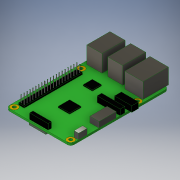
# Autodesk Inventor part: PiB+
Saved by Autodesk Inventor 2016 (Build 200138000, 138)
## iProperties
Created: 2016-08-11
Part Number: PiB+
Material: Generic
Document SubType Name: Modeling
Designer: jfixelle
Density: 1 g/cm^3
Appearance: Smooth - Dark Forest Green
Author: jfixelle
Autodesk Inventor part; units mm, degrees
ref_plane "YZ Plane" through (0, 0, 0) normal (1, 0, 0) x (0, 1, 0)
ref_plane "XZ Plane" through (0, 0, 0) normal (0, 1, 0) x (-1, 0, 0)
ref_plane "XY Plane" through (0, 0, 0) normal (0, 0, 1) x (1, 0, 0)
sketch "Sketch1" plane through (0, 0, 0) normal (0, 1, 0) x (-1, 0, 0)
  line L0 (25, 42.5) -> (-25, 42.5)
  line L1 (-28, 39.5) -> (-28, -39.5)
  line L2 (-25, -42.5) -> (25, -42.5)
  line L3 (28, -39.5) -> (28, 39.5)
  arc A0 (28, 39.5) -> (25, 42.5) centre (25, 39.5) ccw
  arc A1 (25, -42.5) -> (28, -39.5) centre (25, -39.5) ccw
  arc A2 (-28, -39.5) -> (-25, -42.5) centre (-25, -39.5) ccw
  arc A3 (-25, 42.5) -> (-28, 39.5) centre (-25, 39.5) ccw
  line L4 (37.5987, 39) -> (-36.2375, 39) construction
  line L5 (38.7615, -19) -> (-37.8654, -19) construction
  line L6 (-24.5, 52.5969) -> (-24.5, -66.7037) construction
  line L7 (24.5, 56.8992) -> (24.5, -62.5177) construction
  circle A4 centre (24.5, 39) radius 1.4
  circle A5 centre (24.5, -19) radius 1.4
  circle A6 centre (-24.5, -19) radius 1.4
  circle A7 centre (-24.5, 39) radius 1.4
  point P0 (0, 0)
  point P1 (28, 42.5)
  point P2 (-28, -42.5)
  point P3 (28, -42.5)
  dimension "d0" = 85
  dimension "d1" = 56
  dimension "d2" = 42.5
  dimension "d3" = 28
  dimension "d4" = 3
  dimension "d5" = 49
  dimension "d6" = 24.5
  dimension "d7" = 58
  dimension "d8" = 3.5
  dimension "d9" = 2.8
  dimension "d10" = 2.8
  dimension "d11" = 2.8
  dimension "d12" = 2.8
  constraints: 16 end point, 14 point on line, 8 centre point, 8 point on circle, 8 tangent, 3 equal radius, 3 horizontal, 2 parallel, 2 vertical, 1 perpendicular
  measures "d0" distance of point (28, -42.5) point (28, 42.5)
  measures "d1" distance of point (-28, -42.5) point (28, -42.5)
  measures "d2" distance from line of point (0, 0) L2
  measures "d3" distance from line of point (0, 0) L3
  measures "d4" radius of A0
  measures "d5" distance between parallel lines of L6 L7
  measures "d6" distance from line of point (0, 0) L7
  measures "d7" distance between parallel lines of L5 L4
  measures "d8" distance between parallel lines of L0 L4
  measures "d9" diameter of A4
  measures "d10" diameter of A7
  measures "d11" diameter of A6
  measures "d12" diameter of A5
extrude "Extrusion1" add sketch "Sketch1" along normal mid plane 1.65
sketch "Sketch2" plane through (0, 0.825, 0) normal (0, 1, 0) x (1, 0, 0)
  circle A0 centre (-24.5, -39) radius 3.1
  circle A1 centre (-24.5, -39) radius 1.4 projected
  circle A2 centre (-24.5, 19) radius 3.1
  circle A3 centre (24.5, 19) radius 3.1
  circle A4 centre (24.5, -39) radius 3.1
  circle A5 centre (24.5, -39) radius 1.4 projected
  circle A6 centre (24.5, 19) radius 1.4 projected
  circle A7 centre (-24.5, 19) radius 1.4 projected
  point P0 (0, 0)
  dimension "d15" = 6.2
  dimension "d16" = 6.2
  dimension "d17" = 6.2
  dimension "d18" = 6.2
  constraints: 4 centre point, 4 concentric
  measures "d15" diameter of A0
  measures "d16" diameter of A2
  measures "d17" diameter of A3
  measures "d18" diameter of A4
extrude "Extrusion2" add sketch "Sketch2" along normal blind 0.1
mirror "Mirror1" about plane through (0, 0, 0) normal (0, 1, 0) of "Extrusion2"
sketch "Sketch3" plane through (0, 0.825, 0) normal (0, 1, 0) x (1, 0, 0)
  line L0 (-24.5, -35.5) -> (-19.42, -35.5)
  line L1 (-19.42, -35.5) -> (-19.42, 15.3)
  line L2 (-19.42, 15.3) -> (-24.5, 15.3)
  line L3 (-24.5, 15.3) -> (-24.5, -35.5)
  line L4 (-25, -42.5) -> (25, -42.5) projected
  circle A0 centre (-24.5, -39) radius 1.7759
  circle A1 centre (-24.5, -39) radius 1.4 projected
  point P0 (0, 0)
  dimension "d21" = 5.08
  dimension "d22" = 50.8
  dimension "d23" = 7
  dimension "d24" = 0
  constraints: 8 end point, 2 parallel, 1 centre point, 1 concentric, 1 horizontal, 1 perpendicular
  measures "d21" distance of L0.start L0.end
  measures "d22" distance of L0.end L1.end
  measures "d23" distance between parallel lines of L4 L0
  measures "d24" distance from line of A0.centre L3
extrude "Extrusion3" add sketch "Sketch3" along normal blind 1.5 contours L3 L2 L1 L0
sketch "Sketch5" plane through (0, 2.325, 0) normal (0, 1, 0) x (1, 0, 0)
  circle A0 centre (-23.23, -34.23) radius 0.32
  line L0 (-24.5, 15.3) -> (-24.5, -35.5) projected
  line L1 (-24.5, -35.5) -> (-19.42, -35.5) projected
  point P0 (0, 0)
  dimension "d27" = 1.27
  dimension "d28" = 1.27
  dimension "d29" = 0.64
  constraints: 1 centre point
  measures "d27" distance from line of L0 A0.centre
  measures "d28" distance from line of L1 A0.centre
  measures "d29" diameter of A0
extrude "Extrusion4" add sketch "Sketch5" along normal blind 6.1 and the other way blind 4.5
pattern_linear "Rectangular Pattern1" count 20 spacing 2.54 along (0, 0, -1) count 2 spacing 2.54 along (1, 0, 0) of "Extrusion4"
sketch "Sketch6" plane through (0, -0.825, 0) normal (0, -1, 0) x (1, 0, 0)
  line L0 (25, 42.5) -> (-25, 42.5) projected
  line L1 (6.5, 42.5) -> (-8.1, 42.5)
  line L2 (-8.1, 42.5) -> (-8.1, 27.9)
  line L3 (-8.1, 27.9) -> (6.5, 27.9)
  line L4 (6.5, 27.9) -> (6.5, 42.5)
  line L5 (-28, 39.5) -> (-28, -39.5) projected
  line L6 (6.5, 42.5) -> (-8.1, 42.5)
  line L7 (-8.1, 42.5) -> (-8.1, 42.6)
  line L8 (-8.1, 42.6) -> (6.5, 42.6)
  line L9 (6.5, 42.6) -> (6.5, 42.5)
  point P0 (0, 0)
  dimension "d40" = 14.6
  dimension "d41" = 14.6
  dimension "d42" = 19.9
  dimension "d45" = 0.1
  constraints: 16 end point, 4 parallel, 2 horizontal, 2 perpendicular, 1 point on line
  measures "d40" distance of L3.end L1.start
  measures "d41" distance of L2.end L3.end
  measures "d42" distance between parallel lines of L5 L2
  measures "d45" distance between parallel lines of L0 L8
extrude "Extrusion5" add sketch "Sketch6" along normal blind 1.6
sketch "Sketch7" plane through (0, 0.825, 0) normal (0, 1, 0) x (1, 0, 0)
  line L0 (-25, 24.6) -> (-11.9, 24.6)
  line L1 (-11.9, 24.6) -> (-11.9, 44.6)
  line L2 (-11.9, 44.6) -> (-25, 44.6)
  line L3 (-25, 44.6) -> (-25, 24.6)
  line L4 (-7, 24.6) -> (6.1, 24.6)
  line L5 (6.1, 24.6) -> (6.1, 44.6)
  line L6 (6.1, 44.6) -> (-7, 44.6)
  line L7 (-7, 44.6) -> (-7, 24.6)
  line L8 (-28, 39.5) -> (-28, -39.5) projected
  line L9 (-25, -42.5) -> (25, -42.5) projected
  point P0 (0, 0)
  dimension "d46" = 13.1
  dimension "d47" = 13.1
  dimension "d48" = 20
  dimension "d49" = 20
  dimension "d50" = 3
  dimension "d51" = 4.9
  dimension "d52" = 87.1
  dimension "d53" = 0
  constraints: 16 end point, 4 parallel, 2 horizontal, 2 perpendicular
  measures "d46" distance of L1.end L2.end
  measures "d47" distance of L5.end L6.end
  measures "d48" distance of L4.end L5.end
  measures "d49" distance of L0.end L1.end
  measures "d50" distance between parallel lines of L3 L8
  measures "d51" distance between parallel lines of L7 L1
  measures "d52" distance between parallel lines of L9 L2
  measures "d53" distance between parallel lines of L2 L6
extrude "Extrusion6" add sketch "Sketch7" along normal blind 14.8
sketch "Sketch8" plane through (-11.9, 0.825, -44.6) normal (0, 0, -1) x (-1, 0, 0)
  line L0 (-17.45, 12.7988) -> (-5.45, 12.7988)
  line L1 (-5.45, 12.7988) -> (-5.45, 8.2988)
  line L2 (-5.45, 8.2988) -> (-17.45, 8.2988)
  line L3 (-17.45, 8.2988) -> (-17.45, 12.7988)
  line L4 (0.55, 12.7988) -> (12.55, 12.7988)
  line L5 (12.55, 12.7988) -> (12.55, 8.2988)
  line L6 (12.55, 8.2988) -> (0.55, 8.2988)
  line L7 (0.55, 8.2988) -> (0.55, 12.7988)
  line L8 (0.55, 6.5137) -> (12.55, 6.5137)
  line L9 (12.55, 6.5137) -> (12.55, 2.0137)
  line L10 (12.55, 2.0137) -> (0.55, 2.0137)
  line L11 (0.55, 2.0137) -> (0.55, 6.5137)
  line L12 (-17.45, 6.5137) -> (-5.45, 6.5137)
  line L13 (-5.45, 6.5137) -> (-5.45, 2.0137)
  line L14 (-5.45, 2.0137) -> (-17.45, 2.0137)
  line L15 (-17.45, 2.0137) -> (-17.45, 6.5137)
  line L16 (-18, 0) -> (-18, 14.8) projected
  line L17 (0, 0) -> (0, 14.8) projected
  point P0 (-11.9, -0.825)
  dimension "d56" = 12
  dimension "d57" = 12
  dimension "d58" = 12
  dimension "d59" = 12
  dimension "d60" = 0.55
  dimension "d61" = 0.55
  dimension "d62" = 0.55
  dimension "d63" = 0.55
  dimension "d64" = 4.5
  dimension "d65" = 4.5
  dimension "d66" = 4.5
  constraints: 32 end point, 8 parallel, 4 horizontal, 4 perpendicular, 3 point on line
  measures "d56" distance of L0.start L0.end
  measures "d57" distance of L4.start L4.end
  measures "d58" distance of L8.start L8.end
  measures "d59" distance of L12.start L12.end
  measures "d60" distance between parallel lines of L16 L15
  measures "d61" distance between parallel lines of L16 L3
  measures "d62" distance between parallel lines of L17 L7
  measures "d63" distance between parallel lines of L17 L11
  measures "d64" distance of L4.end L5.end
  measures "d65" distance of L8.end L9.end
  measures "d66" distance of L12.end L13.end
extrude "Extrusion7" cut sketch "Sketch8" against normal blind 18
sketch "Sketch9" plane through (-11.9, 0.825, -26.6) normal (0, 0, -1) x (-1, 0, 0)
  line L0 (1.0471, 12.1132) -> (12.1733, 12.1132)
  line L1 (12.1733, 12.1132) -> (12.1733, 10.1863)
  line L2 (12.1733, 10.1863) -> (1.0471, 10.1863)
  line L3 (1.0471, 10.1863) -> (1.0471, 12.1132)
  line L4 (-17.1029, 12.0821) -> (-5.9767, 12.0821)
  line L5 (-5.9767, 12.0821) -> (-5.9767, 10.1553)
  line L6 (-5.9767, 10.1553) -> (-17.1029, 10.1553)
  line L7 (-17.1029, 10.1553) -> (-17.1029, 12.0821)
  line L8 (-17.1029, 5.8975) -> (-5.9767, 5.8975)
  line L9 (-5.9767, 5.8975) -> (-5.9767, 3.9706)
  line L10 (-5.9767, 3.9706) -> (-17.1029, 3.9706)
  line L11 (-17.1029, 3.9706) -> (-17.1029, 5.8975)
  line L12 (1.0471, 5.7732) -> (12.1733, 5.7732)
  line L13 (12.1733, 5.7732) -> (12.1733, 3.8463)
  line L14 (12.1733, 3.8463) -> (1.0471, 3.8463)
  line L15 (1.0471, 3.8463) -> (1.0471, 5.7732)
  point P0 (-11.9, -0.825)
  constraints: 32 end point, 8 parallel, 4 horizontal, 4 perpendicular
extrude "Extrusion8" add sketch "Sketch9" along normal blind 18
sketch "Sketch10" plane through (0, 0.825, 0) normal (0, 1, 0) x (1, 0, 0)
  line L0 (25.7, 22.6) -> (9.8, 22.6)
  line L1 (9.8, 22.6) -> (9.8, 44.6)
  line L2 (9.8, 44.6) -> (25.7, 44.6)
  line L3 (25.7, 44.6) -> (25.7, 22.6)
  line L4 (28, -39.5) -> (28, 39.5) projected
  line L5 (-25, -42.5) -> (25, -42.5) projected
  point P0 (0, 0)
  dimension "d71" = 15.9
  dimension "d72" = 2.3
  dimension "d73" = 22
  dimension "d74" = 87.1
  constraints: 8 end point, 2 parallel, 1 horizontal, 1 perpendicular
  measures "d71" distance of L0.start L0.end
  measures "d72" distance between parallel lines of L4 L3
  measures "d73" distance of L2.end L0.start
  measures "d74" distance between parallel lines of L5 L2
extrude "Extrusion9" add sketch "Sketch10" along normal blind 13.5
sketch "Sketch11" plane through (25.7, 0.825, -44.6) normal (0, 0, -1) x (-1, 0, 0)
  line L0 (2.05, 11.3414) -> (13.85, 11.3414)
  line L1 (13.85, 11.3414) -> (13.85, 4.5414)
  line L2 (13.85, 4.5414) -> (2.05, 4.5414)
  line L3 (2.05, 4.5414) -> (2.05, 11.3414)
  line L4 (4.65, 4.5414) -> (11.25, 4.5414)
  line L5 (11.25, 4.5414) -> (11.25, 2.8514)
  line L6 (11.25, 2.8514) -> (4.65, 2.8514)
  line L7 (4.65, 2.8514) -> (4.65, 4.5414)
  line L8 (0, 0) -> (0, 13.5) projected
  line L9 (7.95, 11.3414) -> (7.95, 4.5414) construction
  point P0 (25.7, -0.825)
  dimension "d77" = 11.8
  dimension "d78" = 2.05
  dimension "d79" = 6.6
  dimension "d80" = 3.3
  dimension "d81" = 6.8
  dimension "d83" = 8.49
  constraints: 18 end point, 4 parallel, 3 perpendicular, 2 horizontal, 2 midpoint, 1 point on line
  measures "d77" distance of L0.start L0.end
  measures "d78" distance between parallel lines of L8 L3
  measures "d79" distance of L5.end L6.end
  measures "d80" distance between parallel lines of L9 L5
  measures "d81" distance of L0.end L1.end
  measures "d83" distance between parallel lines of L6 L0
extrude "Extrusion10" cut sketch "Sketch11" against normal blind 13.5
sketch "Sketch12" plane through (0, 0.825, 0) normal (0, 1, 0) x (1, 0, 0)
  line L0 (20.1, -18) -> (28.1, -18)
  line L1 (28.1, -18) -> (28.1, -3)
  line L2 (28.1, -3) -> (20.1, -3)
  line L3 (20.1, -3) -> (20.1, -18)
  line L4 (24.1, -35.7) -> (28.1, -35.7)
  line L5 (28.1, -35.7) -> (28.1, -28.2)
  line L6 (28.1, -28.2) -> (24.1, -28.2)
  line L7 (24.1, -28.2) -> (24.1, -35.7)
  line L8 (28, 39.5) -> (28, -39.5) projected
  line L9 (15.5, 8) -> (30.5, 8)
  line L10 (30.5, 8) -> (30.5, 14)
  line L11 (30.5, 14) -> (15.5, 14)
  line L12 (15.5, 14) -> (15.5, 8)
  line L13 (-28, 39.5) -> (-28, -39.5) projected
  line L14 (-25, -42.5) -> (25, -42.5) projected
  point P0 (0, 0)
  dimension "d86" = 0.1
  dimension "d87" = 58.5
  dimension "d88" = 6
  dimension "d89" = 15
  dimension "d90" = 7.5
  dimension "d91" = 6.8
  dimension "d92" = 10.2
  dimension "d93" = 11
  dimension "d94" = 4
  dimension "d95" = 8
  dimension "d96" = 15
  constraints: 24 end point, 6 parallel, 3 horizontal, 3 perpendicular, 1 point on line
  measures "d86" distance between parallel lines of L8 L1
  measures "d87" distance between parallel lines of L13 L10
  measures "d88" distance of L11.end L9.start
  measures "d89" distance of L2.end L0.start
  measures "d90" distance of L6.end L4.start
  measures "d91" distance between parallel lines of L14 L4
  measures "d92" distance between parallel lines of L0 L6
  measures "d93" distance between parallel lines of L9 L2
  measures "d94" distance of L5.end L6.end
  measures "d95" distance of L1.end L2.end
  measures "d96" distance of L9.start L9.end
extrude "Extrusion11" add sketch "Sketch12" along normal blind 5
sketch "Sketch13" plane through (0, 0.825, 0) normal (0, 1, 0) x (1, 0, 0)
  line L0 (7.9, 0.5) -> (27.9, 0.5)
  line L1 (27.9, 0.5) -> (27.9, 4.5)
  line L2 (27.9, 4.5) -> (7.9, 4.5)
  line L3 (7.9, 4.5) -> (7.9, 0.5)
  line L4 (-25, -42.5) -> (25, -42.5) projected
  line L5 (28, -3) -> (28, 8) projected
  point P0 (0, 0)
  dimension "d99" = 4
  dimension "d100" = 43
  dimension "d101" = 0.1
  dimension "d102" = 20
  constraints: 8 end point, 2 parallel, 1 horizontal, 1 perpendicular
  measures "d99" distance of L2.end L0.start
  measures "d100" distance between parallel lines of L4 L0
  measures "d101" distance between parallel lines of L5 L1
  measures "d102" distance of L1.end L2.end
extrude "Extrusion12" add sketch "Sketch13" along normal blind 5
sketch "Sketch14" plane through (0, 0.825, 0) normal (0, 1, 0) x (1, 0, 0)
  line L0 (-8.5924, -41.6668) -> (7.5572, -41.6668)
  line L1 (7.5572, -41.6668) -> (7.5572, -38.6911)
  line L2 (7.5572, -38.6911) -> (-8.5924, -38.6911)
  line L3 (-8.5924, -38.6911) -> (-8.5924, -41.6668)
  point P0 (0, 0)
  constraints: 8 end point, 2 parallel, 1 horizontal, 1 perpendicular
extrude "Extrusion13" add sketch "Sketch14" along normal blind 5
sketch "Sketch15" plane through (0, 0.825, 0) normal (0, 1, 0) x (1, 0, 0)
  line L0 (-5.1139, -20.3544) -> (4.8861, -20.3544)
  line L1 (4.8861, -20.3544) -> (4.8861, -10.3544)
  line L2 (4.8861, -10.3544) -> (-5.1139, -10.3544)
  line L3 (-5.1139, -10.3544) -> (-5.1139, -20.3544)
  line L4 (-10.5823, 6.8861) -> (-2.5823, 6.8861)
  line L5 (-2.5823, 6.8861) -> (-2.5823, 14.8861)
  line L6 (-2.5823, 14.8861) -> (-10.5823, 14.8861)
  line L7 (-10.5823, 14.8861) -> (-10.5823, 6.8861)
  point P0 (0, 0)
  dimension "d107" = 8
  dimension "d108" = 8
  dimension "d109" = 10
  dimension "d110" = 10
  constraints: 16 end point, 4 parallel, 2 horizontal, 2 perpendicular
  measures "d107" distance of L6.end L4.start
  measures "d108" distance of L5.end L6.end
  measures "d109" distance of L2.end L0.start
  measures "d110" distance of L1.end L2.end
extrude "Extrusion14" add sketch "Sketch15" along normal blind 1
body "Solid1"
